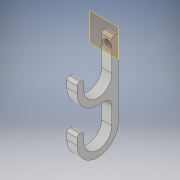
# Autodesk Inventor part: double_rounded_slim
Saved by Autodesk Inventor 2019 (Build 230136000, 136)
## iProperties
Created: 2019-05-03
Part Number: double_rounded_slim
Material: Generic
Document SubType Name: Modeling
Designer: assman
Density: 1 g/cm^3
Appearance: Default
Author: assman
## iProperties of the stored document double_rounded_slim_3DPrint.ipt
Created: 2019-10-22
Part Number: double_rounded_slim_3DPrint
Material: Generic
Document SubType Name: Modeling
Designer: assman
Density: 1 g/cm^3
Appearance: Default
Author: assman
Autodesk Inventor part; units mm, degrees
ref_plane "YZ Plane" through (0, 0, 0) normal (1, 0, 0) x (0, 1, 0)
ref_plane "XZ Plane" through (0, 0, 0) normal (0, 1, 0) x (-1, 0, 0)
ref_plane "XY Plane" through (0, 0, 0) normal (0, 0, 1) x (1, 0, 0)
sketch "Sketch1" plane through (0, 0, 0) normal (1, 0, 0) x (0, 1, 0)
  arc A0 (0, 22) -> (0, 0) centre (0, 11) ccw
  line L0 (-11, 11) -> (24, 11) construction
  arc A1 (35.1478, 22) -> (35.1478, 0) centre (35.1478, 11) ccw
  arc A2 (0, 27) -> (0, -5) centre (0, 11) ccw
  line L1 (0, -5) -> (58, -5)
  arc A3 (35.1478, 5022) -> (35.1478, -5000) centre (35.1478, 11) ccw
  arc A4 (35.1478, 27) -> (19.1478, 11) centre (35.1478, 11) ccw
  line L2 (0, 0) -> (14.1478, 0)
  line L3 (35.1478, 0) -> (58, 0)
  line L4 (35.1478, 27) -> (40.1478, 27)
  line L5 (42.1478, 25) -> (42.1478, 24)
  line L6 (40.1478, 22) -> (35.1478, 22)
  line L7 (0, 27) -> (5, 27)
  line L8 (7, 25) -> (7, 24)
  line L9 (5, 22) -> (0, 22)
  line L10 (60, -2) -> (60, -3)
  arc A5 (40.1478, 22) -> (42.1478, 24) centre (40.1478, 24) ccw
  arc A6 (42.1478, 25) -> (40.1478, 27) centre (40.1478, 25) ccw
  arc A7 (60, -2) -> (58, 0) centre (58, -2) ccw
  arc A8 (58, -5) -> (60, -3) centre (58, -3) ccw
  arc A9 (5, 22) -> (7, 24) centre (5, 24) ccw
  arc A10 (7, 25) -> (5, 27) centre (5, 25) ccw
  line L11 (19.1478, 11) -> (19.1478, 5)
  arc A11 (14.1478, 0) -> (19.1478, 5) centre (14.1478, 5) ccw
  point P0 (60, 0)
  point P1 (42.1478, 27)
  point P2 (42.1478, 22)
  point P3 (7, 27)
  dimension "d0" = 60
  dimension "d1" = 22
  dimension "d2" = 35
  dimension "d3" = 22
  dimension "d5" = 5
  dimension "d6" = 5000
  dimension "d7" = 5
  dimension "d8" = 7
  dimension "d9" = 5
  dimension "d10" = 7
  dimension "d11" = 2
  dimension "d12" = 5
  constraints: 25 point on circle, 24 end point, 19 tangent, 12 centre point, 9 point on line, 5 equal radius, 5 horizontal, 4 perpendicular, 2 vertical
  measures "d0" distance of L2.start point (60, 0)
  measures "d1" distance of L9.end L2.start
  measures "d2" distance of L0.start L0.end
  measures "d3" distance of L3.start L6.end
  measures "d5" radial gap between concentric circles of A0 A2
  measures "d6" radial gap between concentric circles of A1 A3
  measures "d7" radial gap between concentric circles of A1 A4
  measures "d8" distance of L4.start point (42.148, 27)
  measures "d9" distance of point (42.148, 27) point (42.148, 22)
  measures "d10" distance of L7.start point (7, 27)
  measures "d11" radius of A5
  measures "d12" radius of A11
extrude "Extrusion1" add sketch "Sketch1" along normal blind 8
ref_plane "Work Plane1" through (2, 58, 0) normal (0, 0, 1) x (1, 0, 0)
sketch "Sketch2" plane through (2, 58, 0) normal (0, 0, 1) x (1, 0, 0)
  line L0 (-2, 0) -> (6, 0) construction
  line L1 (-2, -22.8522) -> (6, -22.8522) construction
  line L2 (0, 0) -> (4, 0) construction
  line L3 (2, 0) -> (2, -9.8019) construction
  line L4 (-2, 0) -> (-2, -22.8522) projected
  line L5 (6, 0) -> (6, -22.8522) projected
  point P0 (-2, -58)
  point P1 (2, -4.901)
  constraints: 3 midpoint, 2 end point, 1 vertical
hole "Hole1" at (4, 53.099, 0) direction (0, 0, -1) diameter 5 end through all countersink diameter 7 countersink angle 90
body "Solid1"
